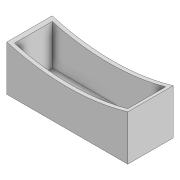
# Autodesk Inventor part: Wasserablauf
Saved by Autodesk Inventor 2021 (Build 250183000, 183)
## iProperties
Created: 2021-09-17
Part Number: Wasserablauf
Material: Generisch
Document SubType Name: Modeling
Designer: lukas
Density: 1 g/cm^3
Appearance: Vorgabe
Author: lukas
Autodesk Inventor part; units mm, degrees
ref_plane "YZ Plane" through (0, 0, 0) normal (1, 0, 0) x (0, 1, 0)
ref_plane "XY Plane" through (0, 0, 0) normal (0, 0, 1) x (1, 0, 0)
sketch "Skizze1" plane through (0, 0, 0) normal (0, 0, 1) x (1, 0, 0)
  line L0 (-56, 0) -> (56, 0) projected
  line L1 (0, -48.0323) -> (0, 183.1937) projected
  line L2 (40, 15) -> (40, -15)
  line L3 (40, -15) -> (-40, -15)
  line L4 (-40, -15) -> (-40, 15)
  arc A0 (-40, 15) -> (40, 15) centre (0, 150.1614) ccw
  point P0 (0, 0)
  dimension "d0" = 80
  constraints: 6 end point, 2 point on circle, 1 centre point, 1 parallel, 1 other
  measures "d0" distance between parallel lines of L2 L4
extrude "Extrusion1" add sketch "Skizze1" against normal blind 30
ref_plane "Arbeitsebene1" through (0, 15, 0) normal (0, 1, 0) x (-1, 0, 0)
sketch "Skizze3" plane through (0, 15, 0) normal (0, 1, 0) x (-1, 0, 0)
  line L0 (37.5, -2.5) -> (-37.5, -2.5)
  line L1 (-37.5, -2.5) -> (-37.5, -27.5)
  line L2 (-37.5, -27.5) -> (37.5, -27.5)
  line L3 (37.5, -27.5) -> (37.5, -2.5)
  line L4 (40, 0) -> (40, -30) projected
  line L5 (40, -30) -> (-40, -30) projected
  line L6 (-40, 0) -> (40, 0) projected
  line L7 (-40, 0) -> (-40, -30) projected
  point P0 (0, 0)
  dimension "d9" = 2.5
  dimension "d10" = 2.5
  dimension "d11" = 2.5
  dimension "d12" = 2.5
  constraints: 8 end point, 2 parallel, 1 horizontal, 1 perpendicular
  measures "d9" distance between parallel lines of L4 L3
  measures "d10" distance between parallel lines of L5 L2
  measures "d11" distance between parallel lines of L6 L0
  measures "d12" distance between parallel lines of L7 L1
extrude "Extrusion2" cut sketch "Skizze3" against normal blind 27.5 contours L3 L2 L1 L0
sketch "Skizze4" plane through (-40, -15, 0) normal (0, -1, 0) x (1, 0, 0)
  line L0 (0, 0) -> (0, -30) projected
  line L1 (80, -30) -> (0, -30) projected
  point P0 (40, 0)
  point P1 (40, -15)
  dimension "d15" = 40
  dimension "d16" = 15
  measures "d15" distance from line of point (40, -15) L0
  measures "d16" distance from line of L1 point (40, -15)
hole "Bohrung1" at (0, -15, -15) direction (0, 1, 0) diameter 9.3762 end through all thread size "M11x1.5" class "6H" standard "ISO Metric profile"
